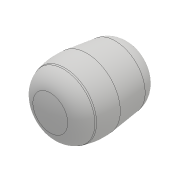
# Autodesk Inventor part: body_ref
Saved by Autodesk Inventor 2017 (Build 210142000, 142)
## iProperties
Created: 2018-06-30
Part Number: body_ref
Material: Generic
Document SubType Name: Modeling
Designer: mfans
Density: 1 g/cm^3
Appearance: Default
Author: mfans
Autodesk Inventor part; units mm, degrees
ref_plane "YZ Plane" through (0, 0, 0) normal (1, 0, 0) x (0, 1, 0)
ref_plane "XZ Plane" through (0, 0, 0) normal (0, 1, 0) x (-1, 0, 0)
ref_plane "XY Plane" through (0, 0, 0) normal (0, 0, 1) x (1, 0, 0)
sketch "Sketch1" plane through (0, 0, 0) normal (0, 0, 1) x (1, 0, 0)
  line L0 (0, 0) -> (40, 0)
  arc A0 (0, -9.4427) -> (40, 0) centre (0, 80) ccw
  line L1 (40, 0) -> (30, 80)
  line L2 (30, 80) -> (0, 80)
  line L3 (0, 80) -> (0, -9.4427)
  dimension "d0" = 40
  dimension "d1" = 80
  dimension "d2" = 30
  constraints: 8 end point, 2 horizontal, 2 point on circle, 1 centre point, 1 perpendicular
  measures "d0" distance of L0.start L0.end
  measures "d1" distance of L0.start L2.end
  measures "d2" distance of L1.end L2.end
revolve "Revolution1" add sketch "Sketch1" angle 360 about axis through (0, 80, 0) along (0, -1, 0)
fillet "Fillet1" radius 20 1 edges at (-30, 80, 0)
chamfer "Chamfer1" distance 10 distance2 20 1 edges at (-40, 0, 0) measured on face at (-36.1941, -1.4854, 7.0791)
fillet "Fillet2" radius 20 1 edges at (-30.8197, -3.9651, 0)
fillet "Fillet3" radius 60 1 edges at (-37.5193, 19.8456, 0)
body "Solid1"
